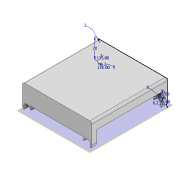
# Autodesk Inventor part: Cage60mm-Boxy
Saved by Autodesk Inventor 2021 (Build 250183000, 183)
## iProperties
Created: 2022-11-30
Part Number: Cage60mm-Boxy
Material: Generic
Document SubType Name: Modeling
Designer: nvladi
Density: 1 g/cm^3
Appearance: Default
Author: nvladi
Autodesk Inventor part; units mm, degrees
ref_plane "YZ Plane" through (0, 0, 0) normal (1, 0, 0) x (0, 1, 0)
ref_plane "XZ Plane" through (0, 0, 0) normal (0, 1, 0) x (-1, 0, 0)
ref_plane "XY Plane" through (0, 0, 0) normal (0, 0, 1) x (1, 0, 0)
sketch "Sketch1" plane through (0, 0, 0) normal (0, 0, 1) x (1, 0, 0)
  arc A0 (-26.899996, 0.000091) -> (-32.192027, -2.19194) centre (-29.999996, 0.000091) ccw
  arc A1 (32.192013, -2.19194) -> (26.899982, 0.000091) centre (29.999982, 0.000091) ccw
  arc A2 (-25.499996, 0.000091) -> (-33.099996, 3.261992) centre (-29.999996, 0.000091) ccw
  arc A3 (33.181962, -3.181889) -> (34.499982, 0.000091) centre (29.999982, 0.000091) ccw
  line L0 (-29.999996, 0.000091) -> (-35.729952, -5.729865)
  line L1 (-29.999996, 0.000091) -> (-21.896614, 0.000091) construction
  line L2 (29.999982, 0.000091) -> (35.185041, -5.184968)
  line L3 (29.999982, 0.000091) -> (37.332763, 0.000091) construction
  line L4 (-29.999996, 0.000091) -> (29.999982, 0.000091)
  line L5 (-34.499996, 0.000255) -> (-34.499996, 20.000255)
  line L6 (-34.499996, 20.000255) -> (34.499982, 20.000255)
  line L7 (34.499982, 20.000255) -> (34.499982, 0.000091)
  line L8 (-31.099996, 18) -> (31.099982, 18)
  line L9 (33.099982, 16) -> (33.099982, 3.261992)
  arc A4 (-33.099996, 3.261992) -> (-34.499996, 0.000091) centre (-29.999996, 0.000091) ccw
  line L10 (-33.099996, 3.261992) -> (-33.099996, 16)
  arc A5 (33.099982, 3.261992) -> (25.499982, 0.000091) centre (29.999982, 0.000091) ccw
  arc A6 (-34.499996, -0.000073) -> (-33.181977, -3.181889) centre (-29.999996, 0.000091) ccw
  arc A7 (-34.499996, 0.000091) -> (-34.499996, -0.000073) centre (-29.999996, 0.000091) ccw
  arc A8 (-33.099996, 7.640683) -> (-29.95922, 4.499906) centre (-30.103466, 7.496437) ccw
  line L11 (-29.95922, 4.499906) -> (-33.099996, 7.640683) construction
  line L12 (-29.95922, 4.499906) -> (-25.517491, 4.499906) construction
  arc A9 (29.959205, 4.499906) -> (33.099982, 7.640683) centre (30.103452, 7.496437) ccw
  line L13 (29.959205, 4.499906) -> (33.099982, 7.640683) construction
  line L14 (29.959205, 4.499906) -> (34.400934, 4.499906) construction
  arc A10 (-31.099996, 18) -> (-33.099996, 16) centre (-31.099996, 16) ccw
  arc A11 (33.099982, 16) -> (31.099982, 18) centre (31.099982, 16) ccw
  point P0 (0, 0)
  point P1 (-33.099996, 18)
  point P2 (33.099982, 18)
  point P3 (-30.164953, 4.497067)
  point P4 (-33.099996, 7.35219)
  point P5 (33.099982, 7.35219)
  point P6 (30.164938, 4.497067)
  dimension "d0" = 6.2
  dimension "d1" = 6.2
  dimension "d2" = 9
  dimension "d3" = 9
  dimension "d4" = 135
  dimension "d5" = 45
  dimension "d6" = 20
  dimension "d17" = 135
  dimension "d18" = 3
  dimension "d19" = 45
  dimension "d20" = 3
  dimension "d23" = 2
  constraints: 31 point on circle, 30 end point, 17 point on line, 12 centre point, 5 horizontal, 4 equal length, 4 tangent, 2 coincident, 1 collinear, 1 equal radius, 1 parallel, 1 perpendicular, 1 vertical
  measures "d0" diameter of A0
  measures "d1" diameter of A1
  measures "d2" diameter of A2
  measures "d3" diameter of A3
  measures "d4" angle of L0 L1
  measures "d5" angle of L2 L3
  measures "d6" distance of L5.start L5.end
  measures "d17" angle of L12 L11
  measures "d18" radius of A8
  measures "d19" angle of L14 L13
  measures "d20" radius of A9
  measures "d23" radius of A10
extrude "Extrusion1" add sketch "Sketch1" along normal blind 75 contours A0 L0 A6 A4 A2 A8 L4 | A8 A2 | A5 A9 L9 A11 L8 A10 L10 A4 L5 L6 L7 A3 L2 A1 L4 | A5 A9
fillet "Fillet1" radius 2 2 edges at (-34.5, 20.0003, 37.5) (34.5, 20.0003, 37.5)
sketch "Sketch1 outline for Extrusion3" plane through (0, 0, 0) normal (0, 0, 1) x (1, 0, 0)
  arc A0 (-30.164953, 4.497067) -> (-33.099996, 7.35219) centre (-30.103466, 7.496437) cw
  arc A1 (-33.099996, 3.261992) -> (-30.164953, 4.497067) centre (-29.999996, 0.000091) cw
  line L0 (-33.099996, 7.35219) -> (-33.099996, 3.261992)
  arc A2 (33.099982, 7.35219) -> (30.164938, 4.497067) centre (30.103452, 7.496437) cw
  line L1 (33.099982, 3.261992) -> (33.099982, 7.35219)
  arc A3 (30.164938, 4.497067) -> (33.099982, 3.261992) centre (29.999982, 0.000091) cw
extrude "Extrusion3" add sketch "Sketch1 outline for Extrusion3" along normal blind 75
ref_plane "Work Plane1" through (-33.099996, -4, 0) normal (0, -1, 0) x (1, 0, 0)
sketch "Sketch2" plane through (-33.099996, -4, 0) normal (0, -1, 0) x (1, 0, 0)
  line L0 (73.099996, 5) -> (-6.900004, 5)
  line L1 (-6.900004, 5) -> (-6.900004, 70)
  line L2 (-6.900004, 70) -> (73.099996, 70)
  line L3 (73.099996, 70) -> (73.099996, 5)
  line L4 (73.099996, 5) -> (-6.900004, 70) construction
  line L5 (-6.900004, 5) -> (73.099996, 70) construction
  point P0 (33.099996, 0)
  point P1 (33.099996, 37.5)
  dimension "d12" = 80
  dimension "d13" = 65
  dimension "d14" = 37.5
  constraints: 12 end point, 2 midpoint, 2 parallel, 1 horizontal, 1 perpendicular
  measures "d12" distance of L1.end L2.end
  measures "d13" distance of L0.end L1.end
  measures "d14" distance of point (33.1, 37.5) point (33.1, 0)
extrude "Extrusion2" cut sketch "Sketch2" against normal blind 15
sketch "Sketch3" plane through (0, 0, 75) normal (0, 0, 1) x (1, 0, 0)
  line L0 (34.499982, 0.000091) -> (34.499982, 18.000255)
  line L1 (-32.499996, 20.000255) -> (32.499982, 20.000255)
  line L2 (34.499982, 18.000255) -> (34.499982, 3.146922)
  line L3 (34.499982, 3.146922) -> (-34.499996, 3.146922)
  line L4 (-34.499996, 3.146922) -> (-34.499996, 18.000255)
  arc A0 (-32.499996, 20.000255) -> (-34.499996, 18.000255) centre (-32.499996, 18.000255) ccw
  arc A1 (34.499982, 18.000255) -> (32.499982, 20.000255) centre (32.499982, 18.000255) ccw
  point P0 (0, 0)
  dimension "d24" = 2
  constraints: 8 end point, 4 point on circle, 4 tangent, 2 centre point, 2 parallel, 1 equal radius, 1 horizontal, 1 perpendicular, 1 point on line
  measures "d24" radius of A0
extrude "Extrusion4" add sketch "Sketch3" against normal blind 2
sketch "Sketch4" plane through (0, 0, 0) normal (0, 0, -1) x (-1, 0, 0)
  line L0 (34.499996, 20.000255) -> (-34.499982, 20.000255)
  line L1 (-34.499982, 20.000255) -> (-34.499982, 0.000091)
  line L2 (34.499996, 0.000255) -> (34.499996, 20.000255)
  line L3 (34.499996, 18.000255) -> (34.499996, 0.000255)
  line L4 (-32.499982, 20.000255) -> (32.499996, 20.000255)
  line L5 (34.499996, 18.000255) -> (34.499996, 3.117372)
  line L6 (34.499996, 3.117372) -> (-34.499982, 3.117372)
  line L7 (-34.499982, 3.117372) -> (-34.499982, 18.000255)
  arc A0 (-32.499982, 20.000255) -> (-34.499982, 18.000255) centre (-32.499982, 18.000255) ccw
  arc A1 (34.499996, 18.000255) -> (32.499996, 20.000255) centre (32.499996, 18.000255) ccw
  point P0 (0, 0)
  point P1 (-34.499982, 3.117372)
  dimension "d27" = 2
  constraints: 8 end point, 4 point on circle, 4 tangent, 3 point on line, 2 centre point, 2 parallel, 1 equal radius, 1 horizontal, 1 perpendicular
  measures "d27" radius of A0
extrude "Extrusion5" add sketch "Sketch4" against normal blind 2 contours A1 L2 L6 L1 A0 L0
body "Solid1"
